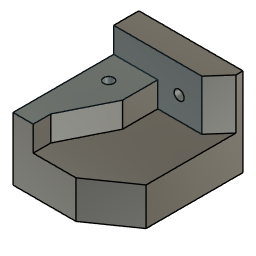
Robocon Task1 a v0 (Autodesk Fusion 360 design; units mm, degrees)
Autodesk Fusion 360 part; units mm, degrees
sketch "Sketch1" plane through (0, 0, 0) normal (0, 0, 1) x (1, 0, 0)
  line L0 (0, 0) -> (0, 50)
  line L1 (0, 0) -> (25, 0)
  line L2 (25, 0) -> (41.383, 11.4715)
  line L3 (25, 0) -> (45, 0) construction
  line L4 (0, 50) -> (41.383, 50)
  line L5 (41.383, 50) -> (41.383, 11.4715)
  dimension "d1" = 50
  dimension "d2" = 25
  dimension "d3" = 35
  dimension "d4" = 20
  constraint coincident L0.start L1.start
  constraint vertical L0
  constraint perpendicular L0 L1
  constraint horizontal L3
  constraint perpendicular L0 L4
  constraint perpendicular L4 L5
  measures "d1" distance of L0.start L0.end
  measures "d2" distance of L0.start L1.end
  measures "d3" angle of L2 L3
  measures "d4" distance of L1.end L2.end
extrude "Extrude1" add sketch "Sketch1" along normal blind 40
extrude "Extrude2" cut 1 faces at (27.5887, 37.1572, 40) along direction (0, 0, -1) blind 25
sketch "Sketch2" plane through (0, 0, 15) normal (0, 0, 1) x (-1, 0, 0)
  line L0 (0, 0) -> (-25, 0)
  line L1 (-25, 0) -> (-41.383, -11.4715)
  line L2 (-41.383, -11.4715) -> (-41.383, -50)
  line L3 (-41.383, -50) -> (0, -50)
  line L4 (0, -50) -> (0, 0)
  line L5 (0, -40) -> (-30, -40)
  line L6 (0, 0) -> (-8, 0)
  line L7 (-8, -15) -> (-8, 0)
  line L8 (-15, -40) -> (-15, -30)
  line L9 (-8, -15) -> (-15, -30)
  line L10 (-30, -40) -> (-35, -40)
  line L11 (-35, -40) -> (-41.383, -47.2262)
  constraint coincident L4 L5.start
  constraint perpendicular L4 L5
  constraint coincident L0.start L4.end
  constraint coincident L0 L6.end
  constraint perpendicular L4 L6
  constraint perpendicular L6 L7
  constraint midpoint L5 L8.start
  constraint perpendicular L5 L8
  constraint parallel L5 L10
  constraint coincident L2 L11.end
extrude "Extrude3" add sketch "Sketch2" along normal blind 20 contours L2 L3 L4 L5 L10 L11
sketch "Sketch3" plane through (0, 0, 15) normal (0, 0, 1) x (-1, 0, 0)
  line L0 (-41.383, -47.2262) -> (-35, -40)
  line L1 (-35, -40) -> (0, -40)
  line L2 (0, -40) -> (0, 0)
  line L3 (0, 0) -> (-25, 0)
  line L4 (-25, 0) -> (-41.383, -11.4715)
  line L5 (-41.383, -11.4715) -> (-41.383, -47.2262)
  line L6 (-17.5, -40) -> (-17.5, -30)
  line L7 (-8, 0) -> (-8, -7)
  line L8 (-17.5, -30) -> (-17.5, -26)
  line L9 (-8, -7) -> (-17.5, -26)
  constraint midpoint L1 L6.start
  constraint perpendicular L1 L6
  constraint coincident L3 L7.start
  constraint perpendicular L3 L7
  constraint perpendicular L1 L8
extrude "Extrude4" add sketch "Sketch3" along normal blind 10 contours L1 L2 L3 L6 L7 L8 L9
sketch "Sketch4" plane through (0, 0, 25) normal (0, 0, 1) x (-1, 0, 0)
  line L0 (-17.5, -40) -> (0, -40)
  line L1 (0, -40) -> (0, 0)
  line L2 (0, 0) -> (-8, 0)
  line L3 (-8, 0) -> (-8, -7)
  line L4 (-8, -7) -> (-17.5, -26)
  line L5 (-17.5, -26) -> (-17.5, -40)
  circle A0 centre (-8, -30) radius 2
extrude "Extrude5" cut sketch "Sketch4" against normal blind 24 contours A0
sketch "Sketch5" plane through (0, 40, 0) normal (0, -1, 0) x (1, 0, 0)
  line L0 (17.5, 25) -> (17.5, 15)
  line L1 (17.5, 15) -> (35, 15)
  line L2 (35, 15) -> (35, 35)
  line L3 (35, 35) -> (0, 35)
  line L4 (0, 35) -> (0, 25)
  line L5 (0, 25) -> (17.5, 25)
sketch "Sketch6" plane through (0, 0, 25) normal (0, 0, 1) x (-1, 0, 0)
  circle A0 centre (-8, -30) radius 2
  line L0 (-17.5, -40) -> (0, -40)
  line L1 (0, -40) -> (0, 0)
  line L2 (0, 0) -> (-8, 0)
  line L3 (-8, 0) -> (-8, -7)
  line L4 (-8, -7) -> (-17.5, -26)
  line L5 (-17.5, -26) -> (-17.5, -40)
sketch "Sketch7" plane through (0, 40, 0) normal (0, -1, 0) x (1, 0, 0)
  circle A0 centre (26, 24) radius 2
  dimension "d17" = 4
  measures "d17" diameter of A0
extrude "Extrude6" cut sketch "Sketch7" against normal blind 8
